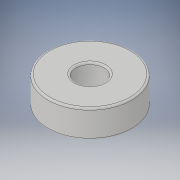
# Autodesk Inventor part: 1614zz bearing
Saved by Autodesk Inventor 2018 (Build 220112000, 112)
## iProperties
Created: 2019-03-22
Part Number: 1614zz bearing
Material: Generic
Document SubType Name: Modeling
Designer: s-4008082
Density: 1 g/cm^3
Appearance: Default
Author: s-4008082
Autodesk Inventor part; units mm, degrees
ref_plane "YZ Plane" through (0, 0, 0) normal (1, 0, 0) x (0, 1, 0)
ref_plane "XZ Plane" through (0, 0, 0) normal (0, 1, 0) x (-1, 0, 0)
ref_plane "XY Plane" through (0, 0, 0) normal (0, 0, 1) x (1, 0, 0)
sketch "Sketch1" plane through (0, 0, 0) normal (0, 1, 0) x (-1, 0, 0)
  circle A0 centre (0, 0) radius 4.7625
  circle A1 centre (0, 0) radius 14.2875
  dimension "d0" = 9.525
  dimension "d1" = 28.575
  constraints: 2 centre point, 2 coincident
  measures "d0" diameter of A0
  measures "d1" diameter of A1
extrude "Extrusion1" add sketch "Sketch1" along normal blind 9.525
fillet "Fillet1" radius 0.635 1 edges at (14.2875, 9.525, 0)
fillet "Fillet2" radius 0.635 1 edges at (14.2875, 0, 0)
fillet "Fillet3" radius 0.635 1 edges at (4.7625, 9.525, 0)
fillet "Fillet4" radius 0.635 1 edges at (4.7625, 0, 0)
body "Solid1"
